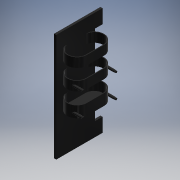
# Autodesk Inventor part: bottom insert
Saved by Autodesk Inventor 2019 (Build 230136000, 136)
## iProperties
Created: 2020-03-05
Part Number: bottom insert
Material: Generic
Document SubType Name: Modeling
Designer: ntb11189
Density: 1 g/cm^3
Appearance: Smooth - Black
Author: ntb11189
Autodesk Inventor part; units mm, degrees
ref_plane "YZ Plane" through (0, 0, 0) normal (1, 0, 0) x (0, 1, 0)
sketch "Sketch1" plane through (0, 0, 0) normal (1, 0, 0) x (0, 1, 0)
  line L0 (0, 0) -> (-116.5, 0)
  line L1 (-116.5, 0) -> (-116.5, -50)
  line L2 (-116.5, -50) -> (0, -50)
  line L3 (0, -50) -> (0, 0)
  dimension "d0" = 116.5
  dimension "d1" = 50
  constraints: 8 end point, 2 parallel, 1 horizontal, 1 perpendicular
  measures "d0" distance of L2.end L1.end
  measures "d1" distance of L0.end L1.end
extrude "Extrusion1" add sketch "Sketch1" along normal blind 2.3
ref_plane "Work Plane1" through (0, -15, 0) normal (0, 1, 0) x (1, 0, 0)
sketch "Sketch5" plane through (0, -15, 0) normal (0, 1, 0) x (1, 0, 0)
  line L0 (-0.3322, 45.1005) -> (1.9678, 45.1005)
  arc A0 (6.7624, 12.7574) -> (17.1624, 12.7574) centre (11.9624, 12.7574) ccw
  line L1 (6.7624, 12.7574) -> (6.7624, 31.3574)
  arc A1 (17.1624, 31.3574) -> (6.7624, 31.3574) centre (11.9624, 31.3574) ccw
  line L2 (17.1624, 31.3574) -> (17.1624, 12.7574)
  line L3 (21.1624, 12.7574) -> (21.1624, 31.3574)
  arc A2 (21.1624, 31.3574) -> (2.7624, 31.3574) centre (11.9624, 31.3574) ccw
  line L4 (2.7624, 31.3574) -> (2.7624, 12.7574)
  arc A3 (2.7624, 12.7574) -> (21.1624, 12.7574) centre (11.9624, 12.7574) ccw
  line L5 (22.4886, 31.3574) -> (22.4886, 12.7574)
  arc A4 (1.4362, 12.7574) -> (22.4886, 12.7574) centre (11.9624, 12.7574) ccw
  line L6 (1.4362, 12.7574) -> (1.4362, 31.3574)
  arc A5 (22.4886, 31.3574) -> (1.4362, 31.3574) centre (11.9624, 31.3574) ccw
  arc A6 (21.6624, 31.3574) -> (2.2624, 31.3574) centre (11.9624, 31.3574) ccw
  line L7 (21.6624, 31.3574) -> (21.6624, 12.7574)
  arc A7 (2.2624, 12.7574) -> (21.6624, 12.7574) centre (11.9624, 12.7574) ccw
  line L8 (2.2624, 12.7574) -> (2.2624, 31.3574)
  point P0 (0, 0)
  point P1 (11.9624, 31.3574)
  dimension "d7" = 0.5
  constraints: 18 end point, 16 point on circle, 8 centre point, 6 other
  measures "d7" radial gap between concentric circles of A2 A6
extrude "Extrusion3" add sketch "Sketch5" against normal blind 10 contours L5 A4 L6 A5
ref_plane "Work Plane2" through (0, -70, 0) normal (0, 1, 0) x (1, 0, 0)
sketch "Sketch6" plane through (0, -70, 0) normal (0, 1, 0) x (1, 0, 0)
  line L0 (2.3, 8.5815) -> (2.3, 11.9041) projected
  arc A0 (2.3, 8.5815) -> (22.4886, 12.7574) centre (11.9624, 12.7574) ccw projected
  line L1 (22.4886, 12.7574) -> (22.4886, 31.3574) projected
  arc A1 (22.4886, 31.3574) -> (2.3, 35.5333) centre (11.9624, 31.3574) ccw projected
  line L2 (2.3, 32.2107) -> (2.3, 35.5333) projected
  arc A2 (21.6624, 31.3574) -> (2.3, 32.2107) centre (11.9624, 31.3574) ccw projected
  line L3 (21.6624, 31.3574) -> (21.6624, 12.7574) projected
  arc A3 (2.3, 11.9041) -> (21.6624, 12.7574) centre (11.9624, 12.7574) ccw projected
  point P0 (0, 0)
extrude "Extrusion4" add sketch "Sketch6" along normal blind 10
sketch "Sketch8" plane through (0, -70, 0) normal (0, -1, 0) x (1, 0, 0)
  line L0 (2.3, -11.9041) -> (2.3, -8.5815) projected
  arc A0 (21.6624, -12.7574) -> (2.3, -11.9041) centre (11.9624, -12.7574) ccw projected
  line L1 (21.6624, -31.3574) -> (21.6624, -12.7574) projected
  arc A1 (2.3, -32.2107) -> (21.6624, -31.3574) centre (11.9624, -31.3574) ccw projected
  line L2 (2.3, -35.5333) -> (2.3, -32.2107) projected
  arc A2 (2.3, -35.5333) -> (22.4886, -31.3574) centre (11.9624, -31.3574) ccw projected
  line L3 (22.4886, -12.7574) -> (22.4886, -31.3574) projected
  arc A3 (22.4886, -12.7574) -> (2.3, -8.5815) centre (11.9624, -12.7574) ccw projected
  line L4 (0, 0) -> (0, -50) projected
  line L5 (0, -50) -> (2.3, -50) projected
  line L6 (2.3, 0) -> (2.3, -50) projected
  line L7 (0, 0) -> (2.3, 0) projected
  line L8 (2.3, -32.2107) -> (2.3, -35.5333) projected
  line L9 (2.3, -11.9041) -> (2.3, -32.2107)
  point P0 (0, 0)
  constraints: 2 end point, 1 collinear
extrude "Extrusion6" add sketch "Sketch8" along normal blind 2 contours L0 A3 L3 A2 L2 A1 L1 A0 | A0 L1 A1 L6
sketch "Sketch9" plane through (22.4886, -60, -12.7574) normal (1, 0, 0) x (0, 0, -1)
  line L0 (0, 45) -> (18.6, 45)
  line L1 (0, 45) -> (0, 35)
  line L2 (18.6, 35) -> (0, 35)
  line L3 (18.6, 45) -> (18.6, 35)
  line L4 (18.6, -12) -> (18.6, 0)
  line L5 (0, 0) -> (18.6, 0)
  line L6 (0, -12) -> (0, 0)
  line L7 (18.6, -12) -> (0, -12)
  line L8 (22.7759, 0) -> (22.7759, -12)
  line L9 (18.6, 0) -> (22.7759, 0)
  line L10 (18.6, -12) -> (18.6, 0)
  line L11 (22.7759, -12) -> (18.6, -12)
  line L12 (0, -12) -> (0, 0)
  line L13 (-4.1759, 0) -> (0, 0)
  line L14 (-4.1759, -12) -> (-4.1759, 0)
  line L15 (0, -12) -> (-4.1759, -12)
  line L16 (-4.1759, 35) -> (-4.1759, 45)
  line L17 (0, 35) -> (-4.1759, 35)
  line L18 (0, 45) -> (0, 35)
  line L19 (-4.1759, 45) -> (0, 45)
  line L20 (22.7759, 45) -> (22.7759, 35)
  line L21 (18.6, 45) -> (22.7759, 45)
  line L22 (18.6, 45) -> (18.6, 35)
  line L23 (22.7759, 35) -> (18.6, 35)
  line L24 (-0.8533, -10) -> (19.4533, -10)
  line L25 (19.4533, -10) -> (19.4533, 0)
  line L26 (19.4533, 0) -> (22.7759, 0)
  line L27 (22.7759, 0) -> (22.7759, -12)
  line L28 (22.7759, -12) -> (-4.1759, -12)
  line L29 (-4.1759, -12) -> (-4.1759, 0)
  line L30 (-4.1759, 0) -> (-0.8533, 0)
  line L31 (-0.8533, 0) -> (-0.8533, -10)
  line L32 (-4.1759, 35) -> (-4.1759, 45)
  line L33 (-4.1759, 45) -> (-0.8533, 45)
  line L34 (-0.8533, 45) -> (-0.8533, 35)
  line L35 (-0.8533, 35) -> (-4.1759, 35)
  line L36 (22.7759, 45) -> (22.7759, 35)
  line L37 (22.7759, 35) -> (19.4533, 35)
  line L38 (19.4533, 35) -> (19.4533, 45)
  line L39 (19.4533, 45) -> (22.7759, 45)
  line L40 (-12.7574, 60) -> (-12.7574, -56.5)
  line L41 (-12.7574, -56.5) -> (37.2426, -56.5)
  line L42 (37.2426, -56.5) -> (37.2426, 60)
  line L43 (37.2426, 60) -> (-12.7574, 60)
  circle A0 centre (26.9827, 18.058) radius 1.25
  circle A1 centre (-8.5773, 18.058) radius 1.25
  circle A2 centre (26.9827, -7.342) radius 1.25
  circle A3 centre (-8.5773, -7.342) radius 1.25
  circle A4 centre (11.7427, -7.342) radius 0.51
  circle A5 centre (9.2027, -7.342) radius 0.51
  circle A6 centre (6.6627, -7.342) radius 0.51
  line L44 (-11.1173, 20.165) -> (-11.1173, -6.882)
  line L45 (-11.1173, -6.882) -> (-11.015, -7.6585)
  line L46 (-11.015, -7.6585) -> (-10.7153, -8.382)
  line L47 (-10.7153, -8.382) -> (-10.2386, -9.0033)
  line L48 (-10.2386, -9.0033) -> (-9.6173, -9.4801)
  line L49 (-9.6173, -9.4801) -> (-8.8937, -9.7798)
  line L50 (-8.8937, -9.7798) -> (-8.1173, -9.882)
  line L51 (-8.1173, -9.882) -> (26.5647, -9.882)
  line L52 (26.5647, -9.882) -> (27.3412, -9.7798)
  line L53 (27.3412, -9.7798) -> (28.0647, -9.4801)
  line L54 (28.0647, -9.4801) -> (28.6861, -9.0033)
  line L55 (28.6861, -9.0033) -> (29.1628, -8.382)
  line L56 (29.1628, -8.382) -> (29.4625, -7.6585)
  line L57 (29.4625, -7.6585) -> (29.5647, -6.882)
  line L58 (29.5647, -6.882) -> (29.5647, 20.165)
  line L59 (29.5647, 20.165) -> (29.4625, 20.9414)
  line L60 (29.4625, 20.9414) -> (29.1628, 21.665)
  line L61 (29.1628, 21.665) -> (28.6861, 22.2863)
  line L62 (28.6861, 22.2863) -> (28.0647, 22.7631)
  line L63 (28.0647, 22.7631) -> (27.3412, 23.0628)
  line L64 (27.3412, 23.0628) -> (26.5647, 23.165)
  line L65 (26.5647, 23.165) -> (-8.1173, 23.165)
  line L66 (-8.1173, 23.165) -> (-8.8937, 23.0628)
  line L67 (-8.8937, 23.0628) -> (-9.6173, 22.7631)
  line L68 (-9.6173, 22.7631) -> (-10.2386, 22.2863)
  line L69 (-10.2386, 22.2863) -> (-10.7153, 21.665)
  line L70 (-10.7153, 21.665) -> (-11.015, 20.9414)
  line L71 (-11.015, 20.9414) -> (-11.1173, 20.165)
  line L72 (29.1262, 0) -> (18.6, 0)
  line L73 (-10.5262, -12) -> (-10.5262, 0)
  line L74 (29.1262, 0) -> (-10.5262, 0)
  line L75 (-10.5262, 0) -> (-10.5262, -12)
  line L76 (-10.5262, -12) -> (29.1262, -12)
  line L77 (29.1262, -12) -> (29.1262, 0)
  point P0 (-11.1173, -9.882)
extrude "Extrusion7" add sketch "Sketch9" against normal up to next contours A2 | A3
sketch "Sketch10" plane through (22.4886, -67.342, -39.7401) normal (1, 0, 0) x (0, 0, -1)
  circle A0 centre (0, 0) radius 1.25 projected
  circle A1 centre (-35.56, 0) radius 1.25 projected
  point P0 (-39.7401, 67.342)
ref_plane "Work Plane3" through (0, -47, 0) normal (0, 1, 0) x (1, 0, 0)
sketch "Sketch11" plane through (0, -47, 0) normal (0, 1, 0) x (1, 0, 0)
  line L0 (2.3, 8.5815) -> (2.3, 11.9041) projected
  arc A0 (2.3, 8.5815) -> (22.4886, 12.7574) centre (11.9624, 12.7574) ccw projected
  line L1 (22.4886, 12.7574) -> (22.4886, 31.3574) projected
  arc A1 (22.4886, 31.3574) -> (2.3, 35.5333) centre (11.9624, 31.3574) ccw projected
  line L2 (2.3, 32.2107) -> (2.3, 35.5333) projected
  arc A2 (21.6624, 31.3574) -> (2.3, 32.2107) centre (11.9624, 31.3574) ccw projected
  line L3 (21.6624, 31.3574) -> (21.6624, 12.7574) projected
  arc A3 (2.3, 11.9041) -> (21.6624, 12.7574) centre (11.9624, 12.7574) ccw projected
  line L4 (0, 50) -> (0, 0) projected
  line L5 (0, 0) -> (2.3, 0) projected
  line L6 (2.3, 50) -> (2.3, 0) projected
  line L7 (0, 50) -> (2.3, 50) projected
extrude "Extrusion9" add sketch "Sketch11" along normal blind 10 contours L0 A3 L3 A2 L2 A1 L1 A0
extrude "Extrusion10" add sketch "Sketch9" against normal up to next contours A0 | A1
extrude "Extrusion11" add sketch "Sketch9" along normal blind 5 contours A0 | A1 | A2 | A3
chamfer "Chamfer1" distance 0.3 distance2 3 1 edges at (27.4886, -67.342, -2.9301) measured on face at (27.4886, -67.4417, -4.5847)
chamfer "Chamfer2" distance 0.3 distance2 3 1 edges at (27.4886, -67.342, -38.4901) measured on face at (27.4886, -67.812, -40.0997)
chamfer "Chamfer3" distance 0.3 distance2 3 1 edges at (27.4886, -41.942, -38.4901) measured on face at (27.4886, -41.6417, -39.2303)
chamfer "Chamfer4" distance 0.3 distance2 3 1 edges at (27.4886, -41.942, -2.9301) measured on face at (27.4886, -42.3316, -4.1328)
sketch "Sketch12" plane through (2.3, 0, 0) normal (1, 0, 0) x (0, 0, -1)
  line L0 (35.5333, -37) -> (35.5333, -47) projected
  line L1 (35.5333, -47) -> (32.2107, -47) projected
  line L2 (32.2107, -47) -> (32.2107, -37) projected
  line L3 (32.2107, -37) -> (35.5333, -37) projected
  line L4 (8.5815, -47) -> (8.5815, -37) projected
  line L5 (8.5815, -37) -> (11.9041, -37) projected
  line L6 (11.9041, -37) -> (11.9041, -47) projected
  line L7 (11.9041, -47) -> (8.5815, -47) projected
  line L8 (11.9041, -70) -> (32.2107, -70) projected
  line L9 (32.2107, -70) -> (32.2107, -60) projected
  line L10 (32.2107, -60) -> (35.5333, -60) projected
  line L11 (35.5333, -60) -> (35.5333, -72) projected
  line L12 (35.5333, -72) -> (8.5815, -72) projected
  line L13 (8.5815, -72) -> (8.5815, -60) projected
  line L14 (8.5815, -60) -> (11.9041, -60) projected
  line L15 (11.9041, -60) -> (11.9041, -70) projected
  line L16 (8.5815, -25) -> (8.5815, -15) projected
  line L17 (8.5815, -15) -> (11.9041, -15) projected
  line L18 (11.9041, -15) -> (11.9041, -25) projected
  line L19 (11.9041, -25) -> (8.5815, -25) projected
  line L20 (35.5333, -15) -> (35.5333, -25) projected
  line L21 (35.5333, -25) -> (32.2107, -25) projected
  line L22 (32.2107, -25) -> (32.2107, -15) projected
  line L23 (32.2107, -15) -> (35.5333, -15) projected
  line L24 (0, 0) -> (0, -116.5) projected
  line L25 (0, -116.5) -> (50, -116.5) projected
  line L26 (50, -116.5) -> (50, 0) projected
  line L27 (50, 0) -> (0, 0) projected
  line L28 (50, -116.5) -> (50, 0) projected
  line L29 (50, -15) -> (42, -15)
  line L30 (42, -15) -> (42, -101.5)
  line L31 (42, -101.5) -> (50, -101.5)
  line L32 (50, -101.5) -> (50, -15)
  dimension "d42" = 8
  dimension "d44" = 15
  dimension "d45" = 15
  constraints: 8 end point, 2 parallel, 1 horizontal, 1 perpendicular, 1 point on line
  measures "d42" distance of L31.end L30.end
  measures "d44" distance between parallel lines of L27 L29
  measures "d45" distance between parallel lines of L25 L31
extrude "Extrusion12" cut sketch "Sketch12" against normal blind 5 contours L26 L31 L30 L29
body "Solid1"
